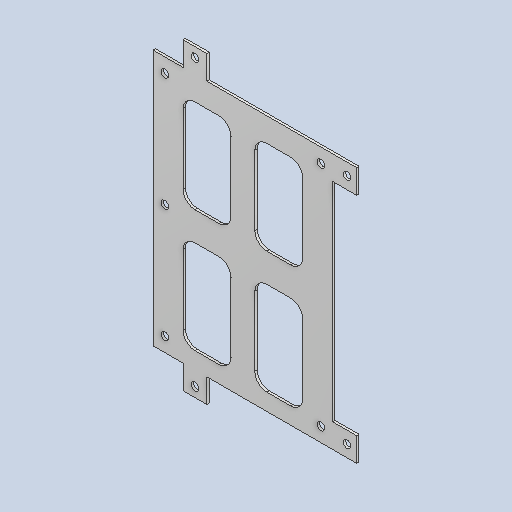
# Autodesk Inventor part: PCB_board_box_left
Saved by Autodesk Inventor 2023 (Build 270158000, 158)
## iProperties
Created: 2023-05-25
Part Number: PCB_board_box_left
Material: Aluminum
Document SubType Name: Sheet Metal
Designer: 310611102
Density: 2.7 g/cm^3
Sheet Metal Rule: Default_mm
Appearance: Satin
Author: 310611102
Autodesk Inventor part; units mm, degrees
ref_plane "YZ Plane" through (0, 0, 0) normal (1, 0, 0) x (0, 1, 0)
ref_plane "XZ Plane" through (0, 0, 0) normal (0, 1, 0) x (-1, 0, 0)
ref_plane "XY Plane" through (0, 0, 0) normal (0, 0, 1) x (1, 0, 0)
sketch "Sketch2" plane through (0, 0, 0) normal (0, 0, 1) x (1, 0, 0)
  line L0 (-37.5, 53.5) -> (37.5, 53.5)
  line L1 (37.5, 53.5) -> (37.5, -53.5)
  line L2 (37.5, -53.5) -> (-37.5, -53.5)
  line L3 (-37.5, -53.5) -> (-37.5, 53.5)
  line L4 (-37.5, 53.5) -> (37.5, -53.5) construction
  line L5 (37.5, 53.5) -> (-37.5, -53.5) construction
  line L6 (-20, 43.5) -> (-10, 43.5)
  line L7 (-5, 38.5) -> (-5, 9.5)
  line L8 (-10, 4.5) -> (-20, 4.5)
  line L9 (-25, 9.5) -> (-25, 38.5)
  line L10 (-25, 43.5) -> (-5, 4.5) construction
  line L11 (-5, 43.5) -> (-25, 4.5) construction
  arc A0 (-20, 43.5) -> (-25, 38.5) centre (-20, 38.5) ccw
  arc A1 (-5, 38.5) -> (-10, 43.5) centre (-10, 38.5) ccw
  arc A2 (-10, 4.5) -> (-5, 9.5) centre (-10, 9.5) ccw
  arc A3 (-25, 9.5) -> (-20, 4.5) centre (-20, 9.5) ccw
  line L12 (10, 43.5) -> (20, 43.5)
  arc A4 (25, 38.5) -> (20, 43.5) centre (20, 38.5) ccw
  arc A5 (20, 4.5) -> (25, 9.5) centre (20, 9.5) ccw
  arc A6 (5, 9.5) -> (10, 4.5) centre (10, 9.5) ccw
  arc A7 (10, 43.5) -> (5, 38.5) centre (10, 38.5) ccw
  line L13 (25, 38.5) -> (25, 9.5)
  line L14 (20, 4.5) -> (10, 4.5)
  line L15 (5, 9.5) -> (5, 38.5)
  line L16 (25, 43.5) -> (5, 4.5) construction
  line L17 (5, 43.5) -> (25, 4.5) construction
  line L18 (-20, -7.5) -> (-10, -7.5)
  arc A8 (-5, -12.5) -> (-10, -7.5) centre (-10, -12.5) ccw
  arc A9 (-10, -46.5) -> (-5, -41.5) centre (-10, -41.5) ccw
  arc A10 (-25, -41.5) -> (-20, -46.5) centre (-20, -41.5) ccw
  arc A11 (-20, -7.5) -> (-25, -12.5) centre (-20, -12.5) ccw
  line L19 (-5, -12.5) -> (-5, -41.5)
  line L20 (-10, -46.5) -> (-20, -46.5)
  line L21 (-25, -41.5) -> (-25, -12.5)
  line L22 (-5, -7.5) -> (-25, -46.5) construction
  line L23 (-25, -7.5) -> (-5, -46.5) construction
  line L24 (10, -7.5) -> (20, -7.5)
  arc A12 (25, -12.5) -> (20, -7.5) centre (20, -12.5) ccw
  arc A13 (20, -46.5) -> (25, -41.5) centre (20, -41.5) ccw
  arc A14 (5, -41.5) -> (10, -46.5) centre (10, -41.5) ccw
  arc A15 (10, -7.5) -> (5, -12.5) centre (10, -12.5) ccw
  line L25 (25, -12.5) -> (25, -41.5)
  line L26 (20, -46.5) -> (10, -46.5)
  line L27 (5, -41.5) -> (5, -12.5)
  line L28 (25, -7.5) -> (5, -46.5) construction
  line L29 (5, -7.5) -> (25, -46.5) construction
  circle A16 centre (-32.6, 0) radius 1.6
  line L30 (0, 0) -> (0, 8.2468)
  circle A17 centre (-32.6, -47.5) radius 1.6
  line L31 (0, 0) -> (-8.4645, 0)
  circle A18 centre (32.6, -47.5) radius 1.6
  circle A19 centre (-32.6, 47.5) radius 1.6
  circle A20 centre (32.6, 47.5) radius 1.6
  point P0 (-15, 24)
  point P1 (15, 24)
  point P2 (-15, -27)
  point P3 (15, -27)
  dimension "d27" = 107
  dimension "d28" = 75
  dimension "d29" = 20
  dimension "d30" = 39
  dimension "d31" = 5
  dimension "d34" = 30
  dimension "d37" = 51
  dimension "d40" = 10
  dimension "d41" = 12.5
  dimension "d42" = 3.2
  dimension "d43" = 4.9
  dimension "d44" = 3.2
  dimension "d45" = 4.9
  dimension "d46" = 6
  measures "d27" distance of L0.end L1.end
  measures "d28" distance of L0.start L0.end
  measures "d29" distance of L10.start L11.start
  measures "d30" distance of L11.end L10.start
  measures "d31" radius of A0
  measures "d34" distance of L6.start L12.start
  measures "d37" distance of L6.start L18.start
  measures "d40" distance between parallel lines of L0 L6
  measures "d41" distance between parallel lines of L3 L9
  measures "d42" diameter of A16
  measures "d43" distance from line of L3 A16.centre
  measures "d44" diameter of A17
  measures "d45" distance from line of L3 A17.centre
  measures "d46" distance from line of L2 A17.centre
sketch "Sketch3" plane through (0, 0, 1) normal (0, 0, 1) x (1, 0, 0)
  arc A0 (25, -12.5) -> (20, -7.5) centre (20, -12.5) ccw
  line L0 (25, -12.5) -> (25, -41.5)
  arc A1 (20, -46.5) -> (25, -41.5) centre (20, -41.5) ccw
  line L1 (20, -46.5) -> (10, -46.5)
  arc A2 (5, -41.5) -> (10, -46.5) centre (10, -41.5) ccw
  line L2 (5, -41.5) -> (5, -12.5)
  arc A3 (10, -7.5) -> (5, -12.5) centre (10, -12.5) ccw
  line L3 (10, -7.5) -> (20, -7.5)
  arc A4 (-5, -12.5) -> (-10, -7.5) centre (-10, -12.5) ccw
  line L4 (-5, -12.5) -> (-5, -41.5)
  arc A5 (-10, -46.5) -> (-5, -41.5) centre (-10, -41.5) ccw
  line L5 (-10, -46.5) -> (-20, -46.5)
  arc A6 (-25, -41.5) -> (-20, -46.5) centre (-20, -41.5) ccw
  line L6 (-25, -41.5) -> (-25, -12.5)
  arc A7 (-20, -7.5) -> (-25, -12.5) centre (-20, -12.5) ccw
  line L7 (-20, -7.5) -> (-10, -7.5)
  arc A8 (25, 38.5) -> (20, 43.5) centre (20, 38.5) ccw
  line L8 (25, 38.5) -> (25, 9.5)
  arc A9 (20, 4.5) -> (25, 9.5) centre (20, 9.5) ccw
  line L9 (20, 4.5) -> (10, 4.5)
  arc A10 (5, 9.5) -> (10, 4.5) centre (10, 9.5) ccw
  line L10 (5, 9.5) -> (5, 38.5)
  arc A11 (10, 43.5) -> (5, 38.5) centre (10, 38.5) ccw
  line L11 (10, 43.5) -> (20, 43.5)
  arc A12 (-20, 43.5) -> (-25, 38.5) centre (-20, 38.5) ccw
  line L12 (-20, 43.5) -> (-10, 43.5)
  arc A13 (-5, 38.5) -> (-10, 43.5) centre (-10, 38.5) ccw
  line L13 (-5, 38.5) -> (-5, 9.5)
  arc A14 (-10, 4.5) -> (-5, 9.5) centre (-10, 9.5) ccw
  line L14 (-10, 4.5) -> (-20, 4.5)
  arc A15 (-25, 9.5) -> (-20, 4.5) centre (-20, 9.5) ccw
  line L15 (-25, 9.5) -> (-25, 38.5)
  circle A16 centre (32.6, 47.5) radius 1.6
  circle A17 centre (-32.6, 47.5) radius 1.6
  circle A18 centre (32.6, -47.5) radius 1.6
  circle A19 centre (-32.6, -47.5) radius 1.6
  circle A20 centre (-32.6, 0) radius 1.6
  line L16 (37.5, 53.5) -> (37.5, -53.5)
  line L17 (-37.5, 53.5) -> (37.5, 53.5)
  line L18 (-37.5, -53.5) -> (-37.5, 53.5)
  line L19 (37.5, -53.5) -> (-37.5, -53.5)
  line L20 (-37.5, 53.5) -> (37.5, 53.5)
  line L21 (-25, 63.5) -> (-15, 63.5)
  line L22 (-15, 63.5) -> (-15, 53.5)
  line L23 (-15, 53.5) -> (-25, 53.5)
  line L24 (-25, 53.5) -> (-25, 63.5)
  line L25 (37.5, 53.5) -> (47.5, 53.5)
  line L26 (47.5, 53.5) -> (47.5, 43.5)
  line L27 (47.5, 43.5) -> (37.5, 43.5)
  line L28 (0, 0) -> (8, 0)
  circle A21 centre (-20, 59.5) radius 1.6
  circle A22 centre (43.5, 48.5) radius 1.6
  line L29 (-25, -63.5) -> (-15, -63.5)
  line L30 (-15, -63.5) -> (-15, -53.5)
  line L31 (-15, -53.5) -> (-25, -53.5)
  line L32 (-25, -53.5) -> (-25, -63.5)
  line L33 (37.5, -53.5) -> (47.5, -53.5)
  line L34 (47.5, -53.5) -> (47.5, -43.5)
  line L35 (47.5, -43.5) -> (37.5, -43.5)
  circle A23 centre (-20, -59.5) radius 1.6
  circle A24 centre (43.5, -48.5) radius 1.6
  line L36 (37.5, 53.5) -> (37.5, 43.5)
  line L37 (37.5, 53.5) -> (37.5, -53.5)
  line L38 (37.5, -53.5) -> (37.5, -43.5)
  point P0 (-20, 63.5)
  point P1 (47.5, 48.5)
  point P2 (-20, -63.5)
  point P3 (47.5, -48.5)
  point P4 (0, 53.5)
  point P5 (0, 53.5)
  dimension "d65" = 4
  dimension "d66" = 10
  dimension "d67" = 10
  dimension "d68" = 10
  dimension "d69" = 10
  dimension "d70" = 4
  dimension "d71" = 3.2
  dimension "d72" = 3.2
  dimension "d77" = 5
  dimension "d78" = 97
  dimension "d79" = 43.5
  dimension "d81" = 119
  dimension "d83" = 20
  dimension "d84" = 12.6
  measures "d65" distance from line of L26 A22.centre
  measures "d66" distance of L25.end L26.end
  measures "d67" distance between parallel lines of L16 L26
  measures "d68" distance of L21.start L21.end
  measures "d69" distance of L21.end L22.end
  measures "d70" distance from line of L21 A21.centre
  measures "d71" diameter of A21
  measures "d72" diameter of A22
  measures "d77" distance from line of L17 A22.centre
  measures "d78" diameter of A22.centre L28
  measures "d79" horizontal distance of A22.centre L28.start
  measures "d81" distance of A23.centre A21.centre
  measures "d83" horizontal distance of A21.centre point (0, 53.5)
  measures "d84" horizontal distance of A21.centre A20.centre
extrude "Plate2" add sketch "Sketch2" along normal blind 1
sheet face with bend "Face3" sketch "Sketch3" thickness 1 toward (0, 0, -1) bend radius 1 contours L25 L26 L27 L16 | L17 L24 L21 L22 | L35 L34 L33 L16 | L30 L29 L32 L19
bend "Bend1"
equation "\"d14\" = 厚度"
equation "\"d53\" = 折彎半徑"
equation "\"d54\" = 折彎離隙寬度"
equation "\"d56\" = 最小剩餘"
equation "\"d55\" = 折彎離隙深度"
equation "\"d57\" = 轉移半徑"
equation "\"折彎半徑\" = 厚度"
equation "\"折彎離隙寬度\" = 厚度"
equation "\"折彎離隙深度\" = 0.5 * 厚度"
equation "\"轉角離隙大小\" = 4 * 厚度"
equation "\"最小剩餘\" = 2 * 厚度"
equation "\"轉移半徑\" = 折彎半徑"
equation "\"Jacobi半徑大小\" = 折彎半徑"
equation "\"間隙大小\" = 厚度"
equation "\"厚度\" = 1"
body "Solid1"
